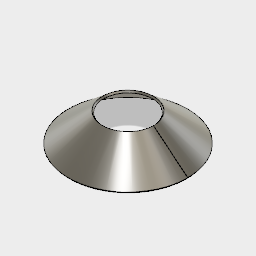
top_roof_actually_used v1 (Autodesk Fusion 360 design; units mm, degrees)
Autodesk Fusion 360 part; units mm, degrees
sketch "スケッチ1" plane through (0, 0, 0) normal (0, 0, 1) x (1, 0, 0)
  line L0 (0, 0) -> (72.5, 0)
  line L1 (0, 0) -> (0, 35)
  line L2 (0, 35) -> (30, 35)
  line L3 (30, 35) -> (72.5, 0)
  line L4 (72.5, 0) -> (74.0893, 1.9298)
  line L5 (74.0893, 1.9298) -> (31.5893, 36.9298)
  line L6 (31.5893, 36.9298) -> (30, 35)
  line L7 (31.5893, 36.9298) -> (0, 36.9298)
  line L8 (31.5893, 36.9298) -> (-4, 42)
  line L9 (31.5893, 36.9298) -> (74.0893, 1.9298)
  line L10 (31.5893, 36.9298) -> (90.0627, 19.4298)
  line L11 (0, 0) -> (0, -10)
  line L12 (0, -10) -> (105, -10)
  line L13 (74.0893, 1.9298) -> (88.5755, -10)
  line L14 (72.5, 0) -> (84.6429, -10)
  dimension "d1" = 72.5
  dimension "d2" = 35
  dimension "d3" = 30
  dimension "d4" = 2.5
  dimension "d5" = 10
  measures "d1" distance of L0.start L0.end
  measures "d2" distance of L0.start L1.end
  measures "d3" distance of L1.end L2.end
  measures "d4" distance of L2.end L5.end
  measures "d5" distance of L0.start L11.end
revolve "回転1" add sketch "スケッチ1" angle 359.9 about axis through (0, 0, 0) along (0, -1, 0) contours L3 L4 L5 L6 L9
extrude "押し出し1" add 1 faces at (45.2261, 24.6199, -0.0789) along direction (0.001745, 0, 0.999998) blind 0.05
